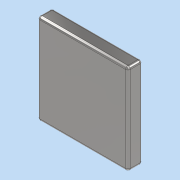
# Autodesk Inventor part: Elektrische Knopf
Saved by Autodesk Inventor 2021 (Build 250183000, 183)
## iProperties
Created: 2024-03-16
Part Number: Elektrische Knopf
Material: Generic
Document SubType Name: Modeling
Designer: Nokia
Density: 1 g/cm^3
Appearance: Galvanized
Author: Nokia
Autodesk Inventor part; units mm, degrees
ref_plane "YZ Plane" through (0, 0, 0) normal (1, 0, 0) x (0, 1, 0)
ref_plane "XZ Plane" through (0, 0, 0) normal (0, 1, 0) x (-1, 0, 0)
ref_plane "XY Plane" through (0, 0, 0) normal (0, 0, 1) x (1, 0, 0)
sketch "Sketch1" plane through (0, 0, 0) normal (0, 0, 1) x (1, 0, 0)
  line L0 (0, 0) -> (150, 0)
  line L1 (150, 0) -> (150, 150)
  line L2 (150, 150) -> (0, 150)
  line L3 (0, 150) -> (0, 0)
  dimension "d0" = 150
  dimension "d1" = 150
  constraints: 8 end point, 3 perpendicular, 1 horizontal
  measures "d0" distance of L0.start L0.end
  measures "d1" distance of L0.end L1.end
extrude "Extrusion1" add sketch "Sketch1" along normal blind 24
fillet "Fillet1" radius 4 12 edges at (75, 150, 24) (75, 150, 0) (150, 75, 0) (150, 75, 24) (0, 75, 0) (0, 75, 24) (75, 0, 24) (75, 0, 0) (0, 0, 12) (150, 0, 12) (150, 150, 12) (0, 150, 12)
body "Solid1"
